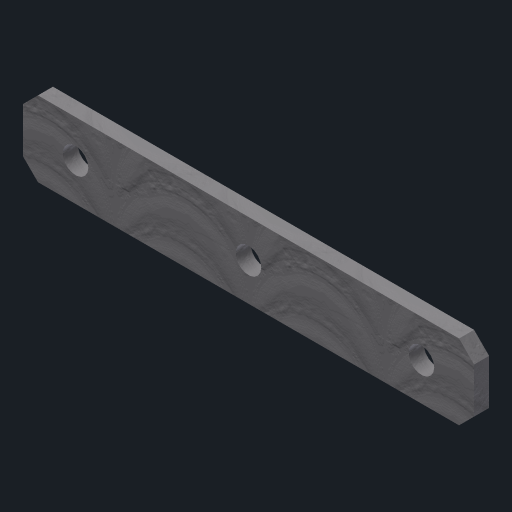
# Autodesk Inventor part: GUIA_DE_AYUDA
Saved by Autodesk Inventor 2024.3 (Build 283343000, 343)
## iProperties
Created: 2024-06-30
Part Number: GUIA_DE_AYUDA
Material: Steel, Mild, Welded
Document SubType Name: Modeling
Designer: Niler
Density: 7.85 g/cm^3
Appearance: Weld - Steel Mild
Author: Niler
Autodesk Inventor part; units mm, degrees
ref_plane "YZ Plane" through (0, 0, 0) normal (1, 0, 0) x (0, 1, 0)
ref_plane "XZ Plane" through (0, 0, 0) normal (0, 1, 0) x (-1, 0, 0)
ref_plane "XY Plane" through (0, 0, 0) normal (0, 0, 1) x (1, 0, 0)
sketch "Sketch1" plane through (0, 0, 0) normal (0, 0, 1) x (1, 0, 0)
  line L0 (-75, -12.5) -> (75, -12.5)
  line L1 (75, -12.5) -> (75, 12.5)
  line L2 (75, 12.5) -> (-75, 12.5)
  line L3 (-75, 12.5) -> (-75, -12.5)
  line L4 (-75, -12.5) -> (75, 12.5) construction
  line L5 (75, -12.5) -> (-75, 12.5) construction
  circle A0 centre (-57.5, 0) radius 4.25
  circle A1 centre (0, 0) radius 4.25
  circle A2 centre (57.5, 0) radius 4.25
  line L6 (-57.5, 0) -> (57.5, 0) construction
  dimension "d0" = 150
  dimension "d1" = 25
  dimension "d3" = 115
  dimension "d4" = 8.5
  constraints: 14 end point, 3 centre point, 3 midpoint, 2 equal radius, 2 horizontal, 2 horizontal alignment, 2 parallel, 1 coincident, 1 perpendicular
  measures "d0" distance of L2.end L1.end
  measures "d1" distance of L1.end L0.end
  measures "d3" distance of L6.end L6.start
  measures "d4" diameter of A0
extrude "Extrusion1" add sketch "Sketch1" along normal blind 5
chamfer "Chamfer1" distance 5 angle 45 4 edges at (-75, 12.5, 2.5) (-75, -12.5, 2.5) (75, -12.5, 2.5) (75, 12.5, 2.5)
body "Solid1"
